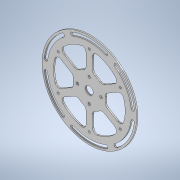
# Autodesk Inventor part: TH22_tire_3rd_POM
Saved by Autodesk Inventor 2022 (Build 260153000, 153)
## iProperties
Created: 2021-11-15
Part Number: TH22_tire_3rd_POM
Material: アルミニウム 6061-AHC
Document SubType Name: Modeling
Designer: 中島 青蔵
Density: 2.7 g/cm^3
Appearance: アルミニウム - ダーク
Author: 中島 青蔵
Autodesk Inventor part; units mm, degrees
ref_plane "YZ Plane" through (0, 0, 0) normal (1, 0, 0) x (0, 1, 0)
ref_plane "XZ Plane" through (0, 0, 0) normal (0, 1, 0) x (-1, 0, 0)
ref_plane "XY Plane" through (0, 0, 0) normal (0, 0, 1) x (1, 0, 0)
sketch "スケッチ1" plane through (0, 0, 0) normal (0, 0, 1) x (1, 0, 0)
  circle A0 centre (0, 0) radius 65
  circle A1 centre (0, 0) radius 55
  circle A2 centre (0, 0) radius 25
  line L0 (0, 0) -> (0, 65)
  circle A3 centre (0, 0) radius 6.05
  line L1 (5, 0) -> (5, 64.8074)
  line L2 (5, 0) -> (69.8074, 0) construction
  line L3 (-5, 0) -> (-5, 64.8074)
  line L4 (-2.5, -4.3301) -> (-58.6249, 28.0736)
  line L5 (2.5, 4.3301) -> (-53.6249, 36.7338)
  line L6 (2.5, -4.3301) -> (-53.6249, -36.7338)
  line L7 (-2.5, 4.3301) -> (-58.6249, -28.0736)
  line L8 (5, 0) -> (5, -64.8074)
  line L9 (-5, 0) -> (-5, -64.8074)
  line L10 (2.5, 4.3301) -> (58.6249, -28.0736)
  line L11 (-2.5, -4.3301) -> (53.6249, -36.7338)
  line L12 (-2.5, 4.3301) -> (53.6249, 36.7338)
  line L13 (2.5, -4.3301) -> (58.6249, 28.0736)
  circle A4 centre (0, 0) radius 72.5
  line L14 (0, 0) -> (36.25, 62.7868)
  line L15 (0, 0) -> (72.5, 0) construction
  line L16 (0, 0) -> (30.6398, 65.7073)
  line L17 (0, 0) -> (72.5, 0) construction
  line L18 (0, 0) -> (41.5843, 59.3885)
  line L19 (0, 0) -> (72.5, 0) construction
  line L20 (0, 65) -> (0, 72.5)
  circle A5 centre (0, 0) radius 69.5
  circle A6 centre (0, 0) radius 64.5
  circle A7 centre (26.0299, 61.7369) radius 2.5
  line L21 (0, 0) -> (-30.6398, 65.7073)
  circle A8 centre (-26.0299, 61.7369) radius 2.5
  circle A9 centre (-40.4507, 53.411) radius 2.5
  circle A10 centre (-66.4807, 8.3259) radius 2.5
  circle A11 centre (-66.4807, -8.3259) radius 2.5
  circle A12 centre (-40.4507, -53.411) radius 2.5
  circle A13 centre (-26.0299, -61.7369) radius 2.5
  circle A14 centre (26.0299, -61.7369) radius 2.5
  circle A15 centre (40.4507, -53.411) radius 2.5
  circle A16 centre (66.4807, -8.3259) radius 2.5
  circle A17 centre (66.4807, 8.3259) radius 2.5
  circle A18 centre (40.4507, 53.411) radius 2.5
  point P0 (5, 54.7723)
  point P1 (44.9342, 31.7163)
  point P2 (18.7132, 16.5776)
  point P3 (5, 24.4949)
  point P4 (-5, 54.7723)
  point P5 (-5, 24.4949)
  point P6 (-18.7132, 16.5776)
  point P7 (-44.9342, 31.7163)
  point P8 (49.9342, -23.056)
  point P9 (23.7132, -7.9173)
  point P10 (23.7132, 7.9173)
  point P11 (49.9342, 23.056)
  point P12 (5, -54.7723)
  point P13 (5, -24.4949)
  point P14 (18.7132, -16.5776)
  point P15 (44.9342, -31.7163)
  point P16 (-44.9342, -31.7163)
  point P17 (-18.7132, -16.5776)
  point P18 (-5, -24.4949)
  point P19 (-5, -54.7723)
  point P20 (-49.9342, 23.056)
  point P21 (-23.7132, 7.9173)
  point P22 (-23.7132, -7.9173)
  point P23 (-49.9342, -23.056)
  point P24 (27.4702, 58.91)
  point P25 (28.2957, 60.6803)
  point P26 (25.0587, 59.4333)
  point P27 (-25.0587, 59.4333)
  point P28 (-28.2957, 60.6803)
  point P29 (-27.4702, 58.91)
  point P30 (-26.6077, 59.3046)
  point P31 (-27.0012, 64.0405)
  point P32 (27.0012, 64.0405)
  point P33 (26.6077, 59.3046)
  point P34 (37.2825, 53.2449)
  point P35 (-64.0001, 8.0152)
  point P36 (-68.9613, 8.6365)
  point P37 (-41.9601, 55.404)
  point P38 (-38.9414, 51.4181)
  point P39 (25.0587, -59.4333)
  point P40 (27.0012, -64.0405)
  point P41 (-27.0012, -64.0405)
  point P42 (-25.0587, -59.4333)
  point P43 (38.9414, 51.4181)
  point P44 (41.9601, 55.404)
  point P45 (68.9613, 8.6365)
  point P46 (64.0001, 8.0152)
  point P47 (64.0001, -8.0152)
  point P48 (68.9613, -8.6365)
  point P49 (41.9601, -55.404)
  point P50 (38.9414, -51.4181)
  point P51 (-38.9414, -51.4181)
  point P52 (-41.9601, -55.404)
  point P53 (-68.9613, -8.6365)
  point P54 (-64.0001, -8.0152)
  dimension "d0" = 130
  dimension "d1" = 110
  dimension "d2" = 50
  dimension "d3" = 12.1
  dimension "d4" = 90
  dimension "d7" = 360
  dimension "d36" = 145
  dimension "d37" = 72.5
  dimension "d38" = 60
  dimension "d39" = 65
  dimension "d40" = 55
  dimension "d41" = 139
  dimension "d42" = 129
  dimension "d43" = 5
  dimension "d50" = 360
  constraints: 44 end point, 19 centre point, 7 coincident, 5 point on circle, 4 equal length, 4 horizontal, 4 symmetric about line, 2 tangent, 63 other
  measures "d0" diameter of A0
  measures "d1" diameter of A1
  measures "d2" diameter of A2
  measures "d3" diameter of A3
  measures "d4" angle of L2 L1
  measures "d36" diameter of A4
  measures "d37" distance of L14.start L14.end
  measures "d38" angle of L15 L14
  measures "d39" angle of L17 L16
  measures "d40" angle of L19 L18
  measures "d41" diameter of A5
  measures "d42" diameter of A6
  measures "d43" diameter of A7
extrude "押し出し1" add sketch "スケッチ1" along normal blind 2 contours A6 L10 A1 L13 | L13 A1 L12 A6 | L12 A1 L18 A6 | A17 A5 A16 A0 | A0 A16 A6 A17 | A5 L18 A4 L21 | L13 A2 L12 A1 | A18 A6 L18 A0 | A0 L18 A18 | A18 L18 A5 | L13 L10 A3 L1 L18 L12 A2 | A2 L10 L13 | L18 A6 L14 A0 | A0 L14 A5 L18 | L18 A1 L14 A6 | L12 L18 A2 | A5 L14 A4 L18 | L10 A6 L11 A1 | A1 L11 A2 L10 | L13 A3 L10 | L10 A2 L11 L8 A3 L13 | L14 A6 L16 A0 | A0 L16 A5 L14 | L14 A1 L16 A6 | L18 L12 L14 A2 | L18 L1 L12 | A5 A14 A0 A15 | A5 L16 A4 L14 | L11 A6 L8 A1 | L16 A6 A7 A0 | A0 A7 L16 | L16 A1 L1 A6 | L14 L1 L16 A2 | L12 L16 L1 | L14 A3 L16 L12 | L1 L18 A3 L14 | L1 A3 L18 | A0 A14 A6 A15 | A5 L20 A4 L16 | L16 A7 A5 | L8 A6 L9 A1 | A1 L9 A2 L8 | A2 L8 L11 | L8 L11 A3 | L1 A2 L0 A1 | A1 L0 A6 L1 | L16 L1 A2 | L16 L12 A3 L0 A2 L1 | L16 A3 L12 | A5 A12 A0 A13 | A4 L20 A5 L21 | L9 A6 L6 A1 | A2 L9 L6 A3 L11 L8 | L0 A2 L3 A1 | A1 L3 A6 L0 | A0 A12 A6 A13 | L21 A0 A9 A5 | A5 A8 L21 | L6 A6 L7 A1 | A1 L7 A2 L6 | A2 L6 L9 | L6 L9 A3 | A1 L21 A6 L3 | L0 A3 L5 L21 L3 A2 | A5 A10 A0 A11 | A8 A0 L21 | L7 A6 L4 A1 | A2 L7 L4 A3 L9 L6 | A1 L5 A6 L21 | L3 L21 A2 | A3 L21 L5 | A0 A10 A6 A11 | L21 A6 A9 A0 | A0 A8 A6 L21 | L4 A6 L5 A1 | A1 L5 A2 L4 | A2 L4 L7 | A3 L3 L5 L21 | L4 L7 A3 | L21 L3 L5 A2 | L21 L5 L3 | A2 L5 L3 A3 L7 L4
sketch "スケッチ2" plane through (0, 0, 2) normal (0, 0, 1) x (1, 0, 0)
  point P0 (0, 0)
  point P1 (0, 18)
  point P2 (-18, 0)
  point P3 (0, -18)
  point P4 (18, 0)
  point P5 (0, 55)
  point P6 (-47.6314, 27.5)
  point P7 (-47.6314, -27.5)
  point P8 (0, -55)
  point P9 (47.6314, -27.5)
  point P10 (47.6314, 27.5)
  dimension "d11" = 18
  dimension "d14" = 360
  dimension "d16" = 55
  dimension "d19" = 360
  constraints: 12 other
  measures "d11" distance of point (0, 0) point (0, 18)
  measures "d16" distance of point (0, 0) point (0, 55)
hole "穴1" at (0, 18, 2) at (-18, 0, 2) at (0, -18, 2) at (18, 0, 2) direction (0, 0, -1) diameter 4 end through all
hole "穴2" at (0, 55, 2) at (-47.6314, 27.5, 2) at (-47.6314, -27.5, 2) at (0, -55, 2) at (47.6314, -27.5, 2) at (47.6314, 27.5, 2) direction (0, 0, -1) diameter 3.2 end through all
fillet "フィレット1" radius 6 24 edges at (-49.9342, 23.056, 1) (-49.9342, -23.056, 1) (-23.7132, -7.9173, 1) (-23.7132, 7.9173, 1) (-44.9342, 31.7163, 1) (-18.7132, 16.5776, 1) (-5, 24.4949, 1) (-5, 54.7723, 1) (5, 54.7723, 1) (5, 24.4949, 1) (18.7132, 16.5776, 1) (44.9342, 31.7163, 1) (49.9342, 23.056, 1) (23.7132, 7.9173, 1) (23.7132, -7.9173, 1) (49.9342, -23.056, 1) (44.9342, -31.7163, 1) (18.7132, -16.5776, 1) (5, -24.4949, 1) (5, -54.7723, 1) (-5, -54.7723, 1) (-5, -24.4949, 1) (-18.7132, -16.5776, 1) (-44.9342, -31.7163, 1)
